split roatry bearing (Autodesk Fusion 360 design; units mm, degrees)
Autodesk Fusion 360 part; units mm, degrees
sketch "Sketch1" plane through (0, 0, 0) normal (0, 0, 1) x (1, 0, 0)
  circle A0 centre (0, 0) radius 15
  circle A1 centre (0, 0) radius 21
  line L0 (20.9914, 0.6) -> (49.9964, 0.6)
  line L1 (49.9964, 0.6) -> (49.9964, -0.6)
  line L2 (49.9964, -0.6) -> (20.9914, -0.6)
  line L3 (20.9914, -0.6) -> (20.9914, 0.6)
  circle A2 centre (0, 0) radius 50
  line L4 (0, 2.5) -> (0, 20)
  line L5 (-49.9964, 0.6) -> (-49.9964, -0.6)
  line L6 (-20.9914, 0.6) -> (-49.9964, 0.6)
  line L7 (-20.9914, -0.6) -> (-20.9914, 0.6)
  line L8 (-49.9964, -0.6) -> (-20.9914, -0.6)
  line L9 (-45.961, 19.6871) -> (-46.4203, 18.5785)
  line L10 (-19.6232, 7.4787) -> (-19.1639, 8.5874)
  line L11 (-46.4203, 18.5785) -> (-19.6232, 7.4787)
  line L12 (-19.1639, 8.5874) -> (-45.961, 19.6871)
  line L13 (19.6232, -7.4787) -> (46.4203, -18.5785)
  line L14 (46.4203, -18.5785) -> (45.961, -19.6871)
  line L15 (19.1639, -8.5874) -> (19.6232, -7.4787)
  line L16 (45.961, -19.6871) -> (19.1639, -8.5874)
  line L17 (-48.1375, 13.5196) -> (-48.4481, 12.3605)
  line L18 (-20.4315, 4.8534) -> (-20.1209, 6.0125)
  line L19 (-48.4481, 12.3605) -> (-20.4315, 4.8534)
  line L20 (-20.1209, 6.0125) -> (-48.1375, 13.5196)
  line L21 (20.4315, -4.8534) -> (48.4481, -12.3605)
  line L22 (48.4481, -12.3605) -> (48.1375, -13.5196)
  line L23 (20.1209, -6.0125) -> (20.4315, -4.8534)
  line L24 (48.1375, -13.5196) -> (20.1209, -6.0125)
  line L25 (-49.4904, 7.1207) -> (-49.647, 5.931)
  line L26 (-20.8902, 2.1451) -> (-20.7335, 3.3348)
  line L27 (-49.647, 5.931) -> (-20.8902, 2.1451)
  line L28 (-20.7335, 3.3348) -> (-49.4904, 7.1207)
  line L29 (20.8902, -2.1451) -> (49.647, -5.931)
  line L30 (49.647, -5.931) -> (49.4904, -7.1207)
  line L31 (20.7335, -3.3348) -> (20.8902, -2.1451)
  line L32 (49.4904, -7.1207) -> (20.7335, -3.3348)
  line L33 (-49.647, -5.931) -> (-49.4904, -7.1207)
  line L34 (-20.7335, -3.3348) -> (-20.8902, -2.1451)
  line L35 (-49.4904, -7.1207) -> (-20.7335, -3.3348)
  line L36 (-20.8902, -2.1451) -> (-49.647, -5.931)
  line L37 (20.7335, 3.3348) -> (49.4904, 7.1207)
  line L38 (49.4904, 7.1207) -> (49.647, 5.931)
  line L39 (20.8902, 2.1451) -> (20.7335, 3.3348)
  line L40 (49.647, 5.931) -> (20.8902, 2.1451)
  line L41 (-48.4481, -12.3605) -> (-48.1375, -13.5196)
  line L42 (-20.1209, -6.0125) -> (-20.4315, -4.8534)
  line L43 (-48.1375, -13.5196) -> (-20.1209, -6.0125)
  line L44 (-20.4315, -4.8534) -> (-48.4481, -12.3605)
  line L45 (20.1209, 6.0125) -> (48.1375, 13.5196)
  line L46 (48.1375, 13.5196) -> (48.4481, 12.3605)
  line L47 (20.4315, 4.8534) -> (20.1209, 6.0125)
  line L48 (48.4481, 12.3605) -> (20.4315, 4.8534)
  line L49 (-46.4203, -18.5785) -> (-45.961, -19.6871)
  line L50 (-19.1639, -8.5874) -> (-19.6232, -7.4787)
  line L51 (-45.961, -19.6871) -> (-19.1639, -8.5874)
  line L52 (-19.6232, -7.4787) -> (-46.4203, -18.5785)
  line L53 (19.1639, 8.5874) -> (45.961, 19.6871)
  line L54 (45.961, 19.6871) -> (46.4203, 18.5785)
  line L55 (19.6232, 7.4787) -> (19.1639, 8.5874)
  line L56 (46.4203, 18.5785) -> (19.6232, 7.4787)
  line L57 (-19.1639, 8.5874) -> (19.1639, 8.5874)
  line L58 (19.1639, -8.5874) -> (-19.1639, -8.5874)
  dimension "d1" = 30
  dimension "d2" = 6
  dimension "d3" = 100
  dimension "d4" = 1.2
  dimension "d6" = 45
  constraint coincident A0.centre A1.centre
  constraint horizontal L0
  constraint vertical L1
  constraint horizontal L2
  constraint vertical L3
  constraint concentric A1 A2
  constraint coincident L0.end A2
  constraint coincident A1 L0.start
  constraint coincident A1 L2.end
  constraint symmetric L0.start L4 L6.start
  constraint symmetric L0.end L4 L5.start
  constraint symmetric L1.end L4 L5.end
  constraint symmetric L2.end L4 L7.start
  measures "d1" diameter of A0
  measures "d2" distance of A0 A1
  measures "d3" diameter of A2
  measures "d4" distance of L0 L2
extrude "Extrude1" add sketch "Sketch1" against normal blind 3 contours A0 L57 L58 | A0 A1 L3 L15 L23 L31 L39 L47 L55 L57 L58 | A1 L53 L54 L56 | A1 L55 | A0 A1 L7 L10 L18 L26 L34 L42 L50 L57 L58 | A1 L15 | A1 L13 L14 L16 | A1 A2 L45 L56 | A1 L10 | A1 L9 L11 L12 | A2 L54 | A1 L49 L51 L52 | A1 L50 | A1 A2 L13 L24 | A2 L14 | A1 L45 L46 L48 | A1 L47 | A1 A2 L11 L20 | A2 L9 | A1 A2 L43 L52 | A2 L49 | A1 L23 | A1 L21 L22 L24 | A1 A2 L37 L48 | A2 L46 | A1 L18 | A1 L17 L19 L20 | A1 L41 L43 L44 | A1 L42 | A1 A2 L21 L32 | A2 L22 | A1 L37 L38 L40 | A1 L39 | A1 A2 L19 L28 | A2 L17 | A1 A2 L35 L44 | A2 L41 | A1 L31 | A1 L29 L30 L32 | A1 L0 A2 L40 | A2 L38 | A1 L26 | A1 L25 L27 L28 | A1 L33 L35 L36 | A1 L34 | A1 L2 A2 L29 | A2 L30 | A1 L0 L1 L2 | A1 L3 | A1 A2 L6 L27 | A2 L25 | A1 A2 L8 L36 | A2 L33 | L1 A2 | A1 L7 | A1 L5 L6 L8 | A2 L5
extrude "Extrude2" add sketch "Sketch1" along normal blind 60 contours A1 L53 L54 L56 | A1 L13 L14 L16 | A1 L9 L11 L12 | A1 L49 L51 L52 | A1 L45 L46 L48 | A1 L21 L22 L24 | A1 L17 L19 L20 | A1 L41 L43 L44 | A1 L37 L38 L40 | A1 L29 L30 L32 | A1 L25 L27 L28 | A1 L33 L35 L36 | A1 L0 L1 L2 | A1 L5 L6 L8
extrude "Extrude3" add sketch "Sketch1" along normal blind 5 from surface at 60 contours A1 L53 L54 L56 | A1 L13 L14 L16 | A1 A2 L45 L56 | A1 L9 L11 L12 | A1 L49 L51 L52 | A1 A2 L13 L24 | A1 L45 L46 L48 | A1 A2 L11 L20 | A1 A2 L43 L52 | A1 L21 L22 L24 | A1 A2 L37 L48 | A1 L17 L19 L20 | A1 L41 L43 L44 | A1 A2 L21 L32 | A1 L37 L38 L40 | A1 A2 L19 L28 | A1 A2 L35 L44 | A1 L29 L30 L32 | A1 L0 A2 L40 | A1 L25 L27 L28 | A1 L33 L35 L36 | A1 L2 A2 L29 | A1 L0 L1 L2 | A1 A2 L6 L27 | A1 A2 L8 L36 | A1 L5 L6 L8
sketch "Sketch2" plane through (0, 0, 65) normal (0, 0, 1) x (-1, 0, 0)
  arc A0 (19.1639, -8.5874) -> (19.1639, 8.5874) centre (0, 0) ccw
  line L0 (19.1639, -8.5874) -> (45.961, -19.6871)
  line L1 (45.961, -19.6871) -> (46.4203, -18.5785)
  arc A1 (46.4203, -18.5785) -> (48.1375, -13.5196) centre (0, 0) ccw
  line L2 (48.1375, -13.5196) -> (48.4481, -12.3605)
  arc A2 (48.4481, -12.3605) -> (49.4904, -7.1207) centre (0, 0) ccw
  line L3 (49.4904, -7.1207) -> (49.647, -5.931)
  arc A3 (49.647, -5.931) -> (49.9964, -0.6) centre (0, 0) ccw
  line L4 (49.9964, -0.6) -> (49.9964, 0.6)
  arc A4 (49.9964, 0.6) -> (49.647, 5.931) centre (0, 0) ccw
  line L5 (49.647, 5.931) -> (49.4904, 7.1207)
  arc A5 (49.4904, 7.1207) -> (48.4481, 12.3605) centre (0, 0) ccw
  line L6 (48.4481, 12.3605) -> (48.1375, 13.5196)
  arc A6 (48.1375, 13.5196) -> (46.4203, 18.5785) centre (0, 0) ccw
  line L7 (46.4203, 18.5785) -> (45.961, 19.6871)
  line L8 (45.961, 19.6871) -> (19.1639, 8.5874)
  line L9 (-45.961, 19.6871) -> (-46.4203, 18.5785)
  arc A7 (-46.4203, 18.5785) -> (-48.1375, 13.5196) centre (0, 0) ccw
  line L10 (-48.1375, 13.5196) -> (-48.4481, 12.3605)
  arc A8 (-48.4481, 12.3605) -> (-49.4904, 7.1207) centre (0, 0) ccw
  line L11 (-49.4904, 7.1207) -> (-49.647, 5.931)
  arc A9 (-49.647, 5.931) -> (-49.9964, 0.6) centre (0, 0) ccw
  line L12 (-49.9964, 0.6) -> (-49.9964, -0.6)
  arc A10 (-49.9964, -0.6) -> (-49.647, -5.931) centre (0, 0) ccw
  line L13 (-49.647, -5.931) -> (-49.4904, -7.1207)
  arc A11 (-49.4904, -7.1207) -> (-48.4481, -12.3605) centre (0, 0) ccw
  line L14 (-48.4481, -12.3605) -> (-48.1375, -13.5196)
  arc A12 (-48.1375, -13.5196) -> (-46.4203, -18.5785) centre (0, 0) ccw
  line L15 (-46.4203, -18.5785) -> (-45.961, -19.6871)
  line L16 (-45.961, -19.6871) -> (-19.1639, -8.5874)
  arc A13 (-19.1639, -8.5874) -> (-19.1639, 8.5874) centre (0, 0) cw
  line L17 (-19.1639, 8.5874) -> (-45.961, 19.6871)
  line L18 (19.1639, -8.5874) -> (-19.1639, -8.5874)
  line L19 (-19.1639, -8.5874) -> (-19.1639, 8.5874)
  line L20 (-19.1639, 8.5874) -> (19.1639, 8.5874)
  line L21 (19.1639, 8.5874) -> (19.1639, -8.5874)
  constraint horizontal L18
  constraint vertical L19
  constraint horizontal L20
  constraint vertical L21
  constraint coincident A13.end L17.start
  constraint coincident A0.start L0.start
extrude "Extrude4" add sketch "Sketch2" along normal blind 3
chamfer "Chamfer1" distance 2.943 angle 45 2 edges at (-21, 0, 65) (21, 0, 65)
